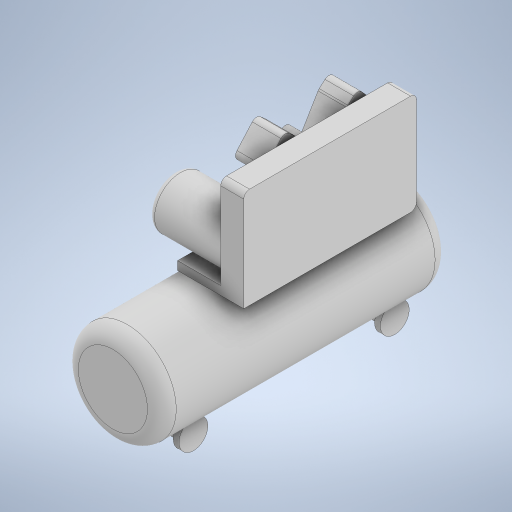
# Autodesk Inventor part: compressor
Saved by Autodesk Inventor 2023.1 (Build 271208000, 208)
## iProperties
Created: 2023-08-14
Part Number: compressor
Material: Generic
Document SubType Name: Modeling
Designer: admin
Density: 1 g/cm^3
Appearance: Default
Author: admin
Autodesk Inventor part; units mm, degrees
ref_plane "YZ Plane" through (0, 0, 0) normal (1, 0, 0) x (0, 1, 0)
ref_plane "XZ Plane" through (0, 0, 0) normal (0, 1, 0) x (-1, 0, 0)
ref_plane "XY Plane" through (0, 0, 0) normal (0, 0, 1) x (1, 0, 0)
sketch "Sketch2" plane through (0, 0, 0) normal (0, 0, 1) x (1, 0, 0)
  circle A0 centre (0, 220) radius 170
  point P0 (0, 0)
  dimension "d1" = 340
  dimension "d2" = 220
  constraints: 1 centre point, 1 vertical alignment
  measures "d1" diameter of A0
  measures "d2" distance of point (0, 0) A0.centre
extrude "Extrusion1" add sketch "Sketch2" along normal mid plane 1000
sketch "Sketch3" plane through (0, 0, 0) normal (1, 0, 0) x (0, 1, 0)
  line L0 (50, -500) -> (390, -500) projected
  line L1 (390, 500) -> (50, 500) projected
  circle A0 centre (510, 110) radius 90
  line L2 (390, -500) -> (390, 500) projected
  line L3 (390, 200) -> (420, 200)
  line L4 (420, 200) -> (420, -350)
  line L5 (420, -350) -> (390, -350)
  line L6 (390, -350) -> (390, 200)
  line L7 (390, 0) -> (807.84, 0) construction
  line L8 (510, 20) -> (580, 20) construction
  line L9 (420, -175) -> (650, -175)
  line L10 (650, -175) -> (560, -255)
  line L11 (560, -255) -> (420, -275)
  line L12 (650, -175) -> (560, -95)
  line L13 (560, -95) -> (420, -75)
  arc A1 (633.1833, -189.9482) -> (633.1833, -160.0518) centre (619.896, -175) ccw
  point P0 (0, 0)
  point P1 (420, 110)
  dimension "d5" = 180
  dimension "d6" = 150
  dimension "d7" = 300
  dimension "d8" = 30
  dimension "d9" = 70
  dimension "d10" = 20
  dimension "d12" = 230
  dimension "d13" = 160
  dimension "d14" = 200
  dimension "d15" = 140
  dimension "d16" = 20
  constraints: 22 end point, 6 point on line, 3 midpoint, 3 parallel, 3 perpendicular, 2 equal length, 2 horizontal, 2 point on circle, 2 tangent, 1 centre point, 1 vertical, 5 other
  measures "d6" distance between parallel lines of L5 L0
  measures "d7" distance between parallel lines of L3 L1
  measures "d8" distance of L3.start L3.end
  measures "d9" distance of L8.start L8.end
  measures "d10" distance between parallel lines of L7 L8
  measures "d12" distance of L9.start L9.end
  measures "d13" distance of L10.end L12.end
  measures "d14" distance of L11.end L13.end
  measures "d15" distance from line of L4 L10.end
  measures "d16" radius of A1
extrude "Extrusion2" add sketch "Sketch3" along normal mid plane 150 contours A0 | L4 L5 L2 L3 | L13 L12 A1 L9 L4 | L9 A1 L10 L11 L4
sketch "Sketch4" plane through (-75, 510, 110) normal (-1, 0, 0) x (0, 0, 1)
  circle A0 centre (0, 0) radius 90 projected
  point P0 (-110, -510)
  point P1 (0, -90)
  constraints: 1 vertical alignment
extrude "Extrusion3" add sketch "Sketch4" along normal blind 100
sketch "Sketch5" plane through (75, 0, 0) normal (1, 0, 0) x (0, 0, -1)
  line L0 (500, 390) -> (-500, 390) projected
  line L1 (-200, 740) -> (400, 740)
  line L2 (400, 740) -> (400, 390)
  line L3 (400, 390) -> (-200, 390)
  line L4 (-200, 390) -> (-200, 740)
  line L5 (500, 50) -> (500, 390) projected
  point P0 (0, 0)
  dimension "d21" = 600
  dimension "d22" = 350
  dimension "d23" = 100
  constraints: 8 end point, 2 parallel, 1 horizontal, 1 perpendicular, 1 point on line
  measures "d21" distance of L1.start L1.end
  measures "d22" distance of L3.end L1.start
  measures "d23" distance between parallel lines of L2 L5
extrude "Extrusion4" add sketch "Sketch5" along normal blind 80
sketch "Sketch6" plane through (0, 0, 0) normal (1, 0, 0) x (0, 1, 0)
  line L0 (420, -275) -> (420, -350) projected
  line L1 (420, -350) -> (390, -350) projected
  line L2 (390, -350) -> (390, 200) projected
  line L3 (390, 200) -> (420, 200) projected
  line L4 (420, 200) -> (420, 110) projected
  line L5 (420, 110) -> (420, -75) projected
  line L6 (420, -75) -> (560, -95) projected
  line L7 (560, -95) -> (633.1833, -160.0518) projected
  arc A0 (633.1833, -189.9482) -> (633.1833, -160.0518) centre (619.896, -175) ccw projected
  line L8 (633.1833, -189.9482) -> (560, -255) projected
  line L9 (560, -255) -> (420, -275) projected
  line L10 (633.1833, -160.0518) -> (560, -95) projected
  line L11 (596.5916, -127.5259) -> (702.8899, -7.9404)
  line L12 (560, -255) -> (633.1833, -189.9482) projected
  line L13 (619.896, -175) -> (390, -175) construction
  line L14 (390, 200) -> (390, -400) projected
  line L15 (747.7344, -47.8022) -> (658.0453, 31.9214)
  line L16 (747.7344, -47.8022) -> (714.5162, -85.1727)
  line L17 (658.0453, 31.9214) -> (624.8271, -5.4491)
  line L18 (624.8271, -5.4491) -> (577.9064, -110.9168)
  line L19 (714.5162, -85.1727) -> (615.2769, -144.135)
  line L20 (596.5916, -222.4741) -> (702.8899, -342.0596)
  line L21 (747.7344, -302.1978) -> (658.0453, -381.9214)
  line L22 (747.7344, -302.1978) -> (714.5162, -264.8273)
  line L23 (658.0453, -381.9214) -> (624.8271, -344.5509)
  line L24 (624.8271, -344.5509) -> (577.9064, -239.0832)
  line L25 (714.5162, -264.8273) -> (615.2769, -205.865)
  point P0 (0, 0)
  dimension "d26" = 160
  dimension "d27" = 120
  dimension "d28" = 50
  dimension "d29" = 50
  constraints: 26 end point, 8 symmetric about line, 5 perpendicular, 3 midpoint, 3 point on line, 2 equal length
  measures "d26" distance of L11.end L11.start
  measures "d27" distance of L15.start L15.end
  measures "d28" distance of L15.start L16.end
  measures "d29" distance of L18.end L19.end
extrude "Extrusion5" add sketch "Sketch6" along normal mid plane 100 contours L8 L20 L21 L23 L24 | L8 L25 L22 L21 L20 | L7 L11 L15 L16 L19 | L18 L17 L15 L11 L7
fillet "Fillet1" radius 50 2 edges at (-170, 220, -500) (-170, 220, 500)
fillet "Fillet2" radius 20 1 edges at (-175, 510, 20)
fillet "Fillet3" radius 20 8 edges at (0, 747.7344, -302.1978) (0, 658.0453, -381.9214) (0, 747.7344, -47.8022) (0, 658.0453, 31.9214) (0, 714.5162, -85.1727) (0, 624.8271, -5.4491) (0, 714.5162, -264.8273) (0, 624.8271, -344.5509)
fillet "Fillet4" radius 20 3 edges at (115, 740, -400) (115, 740, 200) (115, 390, -400)
sketch "Sketch7" plane through (0, 0, 0) normal (1, 0, 0) x (0, 1, 0)
  line L0 (50, -450) -> (50, 450) projected
  line L1 (50, -400) -> (30, -400)
  line L2 (30, -400) -> (30, -350)
  line L3 (30, -350) -> (50, -350)
  line L4 (50, -350) -> (50, -400)
  line L5 (50, 300) -> (30, 300)
  line L6 (30, 300) -> (30, 350)
  line L7 (30, 350) -> (50, 350)
  line L8 (50, 350) -> (50, 300)
  point P0 (0, 0)
  dimension "d36" = 50
  dimension "d37" = 350
  dimension "d38" = 300
  dimension "d39" = 20
  constraints: 16 end point, 4 parallel, 3 point on line, 2 horizontal, 2 perpendicular, 1 collinear
  measures "d36" distance of L1.end L2.end
  measures "d37" distance from line of point (0, 0) L3
  measures "d38" distance from line of point (0, 0) L5
  measures "d39" distance of L1.start L1.end
extrude "Extrusion6" add sketch "Sketch7" along normal mid plane 170
sketch "Sketch8" plane through (-85, 0, 0) normal (-1, 0, 0) x (0, 0, 1)
  line L0 (-400, 50) -> (-400, 30) projected
  line L1 (-400, 30) -> (-350, 30) projected
  line L2 (-350, 30) -> (-350, 50) projected
  line L3 (-350, 50) -> (-400, 50) projected
  line L4 (300, 50) -> (300, 30) projected
  line L5 (300, 30) -> (350, 30) projected
  line L6 (350, 30) -> (350, 50) projected
  line L7 (350, 50) -> (300, 50) projected
  line L8 (-350, 50) -> (-400, 50) projected
  circle A0 centre (-375, 50) radius 50
  line L9 (350, 50) -> (300, 50) projected
  circle A1 centre (325, 50) radius 50
  point P0 (0, 0)
  dimension "d42" = 100
  constraints: 2 centre point, 2 midpoint, 1 equal radius
  measures "d42" diameter of A0
extrude "Extrusion7" add sketch "Sketch8" along normal blind 20 contours L3 L2 L1 L0 | L7 L6 L5 L4 | A0 | A1
mirror "Mirror1" about plane through (0, 0, 0) normal (1, 0, 0) of "Extrusion7"
body "Solid1"
